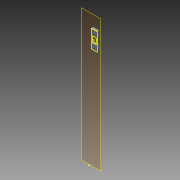
# Autodesk Inventor part: boardHolderv2
Saved by Autodesk Inventor 2014 (Build 180170000, 170)
## iProperties
Created: 2014-01-11
Part Number: boardHolderv2
Material: Generic
Document SubType Name: Modeling
Designer: intern
Density: 1 g/cm^3
Appearance: Default
Author: intern
Autodesk Inventor part; units mm, degrees
ref_plane "YZ Plane" through (0, 0, 0) normal (1, 0, 0) x (0, 1, 0)
ref_plane "XZ Plane" through (0, 0, 0) normal (0, 1, 0) x (-1, 0, 0)
ref_plane "XY Plane" through (0, 0, 0) normal (0, 0, 1) x (1, 0, 0)
ref_plane "Work Plane1" through (0, 0, 0) normal (0, 0, 1) x (1, 0, 0)
sketch "Sketch1" plane through (0, 0, 0) normal (0, 0, 1) x (1, 0, 0)
  circle A0 centre (26.9875, 590.55) radius 15.621 projected
  line L0 (11.3665, 606.171) -> (42.6085, 606.171)
  line L1 (42.6085, 606.171) -> (42.6085, 574.929)
  line L2 (42.6085, 574.929) -> (11.3665, 574.929)
  line L3 (11.3665, 574.929) -> (11.3665, 606.171)
  line L4 (11.3665, 606.171) -> (42.6085, 574.929) construction
  line L5 (42.6085, 606.171) -> (11.3665, 574.929) construction
  line L6 (10.8585, 637.921) -> (43.1165, 637.921)
  line L7 (43.1165, 637.921) -> (43.1165, 543.179)
  line L8 (43.1165, 543.179) -> (10.8585, 543.179)
  line L9 (10.8585, 543.179) -> (10.8585, 637.921)
  line L10 (10.8585, 637.921) -> (43.1165, 543.179) construction
  line L11 (43.1165, 637.921) -> (10.8585, 543.179) construction
  line L12 (42.6085, 606.171) -> (43.1165, 606.171)
  line L13 (11.3665, 606.171) -> (10.8585, 606.171)
  line L14 (11.3665, 574.929) -> (10.8585, 574.929)
  line L15 (42.6085, 574.929) -> (43.1165, 574.929)
  point P0 (0, 0)
  dimension "d0" = 32.258
  dimension "d1" = 94.742
  constraints: 32 end point, 5 equal length, 5 perpendicular, 4 midpoint, 4 point on line, 3 horizontal, 1 vertical
  measures "d0" distance of L7.end L8.end
  measures "d1" distance of L6.end L7.end
extrude "Extrusion1" add sketch "Sketch1" along normal blind 5.08 contours L0 L13 L9 L6 L7 L12 | L2 L15 L7 L8 L9 L14
sketch "Sketch2" plane through (0, 0, 5.08) normal (0, 0, 1) x (1, 0, 0)
  line L0 (10.8585, 606.171) -> (43.1165, 606.171) projected
  line L1 (43.1165, 606.171) -> (43.1165, 637.921) projected
  line L2 (43.1165, 637.921) -> (10.8585, 637.921) projected
  circle A0 centre (26.9875, 590.55) radius 8.9481 projected
  line L3 (35.8299, 591.9213) -> (35.0382, 597.0264) projected
  line L4 (35.0382, 597.0264) -> (30.2211, 598.8934) projected
  line L5 (36.6216, 586.8161) -> (35.8299, 591.9213) projected
  line L6 (32.5963, 583.5779) -> (36.6216, 586.8161) projected
  line L7 (28.5709, 580.3397) -> (32.5963, 583.5779) projected
  line L8 (23.7539, 582.2066) -> (28.5709, 580.3397) projected
  line L9 (28.1112, 583.3043) -> (33.8243, 587.9003) projected
  line L10 (33.8243, 587.9003) -> (32.7007, 595.146) projected
  line L11 (32.7007, 595.146) -> (25.8638, 597.7957) projected
  line L12 (25.8638, 597.7957) -> (20.1507, 593.1997) projected
  line L13 (20.1507, 593.1997) -> (21.2743, 585.954) projected
  line L14 (21.2743, 585.954) -> (28.1112, 583.3043) projected
  line L15 (28.5709, 580.3397) -> (18.9368, 584.0736) projected
  line L16 (18.9368, 584.0736) -> (17.3534, 594.2839) projected
  line L17 (17.3534, 594.2839) -> (25.4041, 600.7603) projected
  line L18 (25.4041, 600.7603) -> (35.0382, 597.0264) projected
  line L19 (35.0382, 597.0264) -> (36.6216, 586.8161) projected
  line L20 (36.6216, 586.8161) -> (28.5709, 580.3397) projected
  line L21 (43.1165, 574.929) -> (10.8585, 574.929) projected
  line L22 (10.8585, 574.929) -> (10.8585, 543.179) projected
  line L23 (10.8585, 543.179) -> (43.1165, 543.179) projected
  line L24 (43.1165, 543.179) -> (43.1165, 574.929) projected
  line L25 (43.1165, 637.921) -> (37.3198, 637.921)
  line L26 (37.3198, 543.179) -> (43.1165, 543.179)
  line L27 (43.1165, 543.179) -> (43.1165, 637.921)
  line L28 (10.8585, 543.179) -> (16.6552, 543.179)
  line L29 (16.6552, 637.921) -> (10.8585, 637.921)
  line L30 (10.8585, 637.921) -> (10.8585, 543.179)
  line L31 (37.3198, 637.921) -> (16.6552, 637.921)
  line L32 (16.6552, 637.921) -> (16.6552, 606.171)
  line L33 (16.6552, 606.171) -> (37.3198, 606.171)
  line L34 (37.3198, 606.171) -> (37.3198, 637.921)
  line L35 (37.3198, 574.929) -> (16.6552, 574.929)
  line L36 (16.6552, 574.929) -> (16.6552, 543.179)
  line L37 (16.6552, 543.179) -> (37.3198, 543.179)
  line L38 (37.3198, 543.179) -> (37.3198, 574.929)
  circle A1 centre (26.9875, 590.55) radius 10.9728
  line L39 (37.3198, 606.171) -> (37.3198, 594.2439)
  line L40 (37.3198, 586.8561) -> (37.3198, 574.929)
  line L41 (43.1165, 637.921) -> (43.1165, 543.179)
  line L42 (43.1165, 543.179) -> (37.3198, 543.179)
  line L43 (37.3198, 637.921) -> (43.1165, 637.921)
  line L44 (16.6552, 637.921) -> (16.6552, 594.2439)
  line L45 (16.6552, 586.8561) -> (16.6552, 543.179)
  line L46 (10.8585, 543.179) -> (43.1165, 543.179)
  line L47 (43.1165, 543.179) -> (43.1165, 574.929)
  line L48 (43.1165, 574.929) -> (10.8585, 574.929)
  line L49 (10.8585, 574.929) -> (10.8585, 543.179)
  line L50 (10.8585, 637.921) -> (43.1165, 637.921)
  line L51 (43.1165, 637.921) -> (43.1165, 606.171)
  line L52 (43.1165, 606.171) -> (10.8585, 606.171)
  line L53 (10.8585, 606.171) -> (10.8585, 637.921)
  line L54 (16.6552, 574.929) -> (10.8585, 574.929)
  line L55 (10.8585, 574.929) -> (10.8585, 543.179)
  line L56 (10.8585, 543.179) -> (16.6552, 543.179)
  line L57 (16.6552, 543.179) -> (16.6552, 574.929)
  line L58 (43.1165, 574.929) -> (37.3198, 574.929)
  line L59 (37.3198, 574.929) -> (37.3198, 543.179)
  line L60 (37.3198, 543.179) -> (43.1165, 543.179)
  line L61 (43.1165, 543.179) -> (43.1165, 574.929)
  line L62 (16.6552, 586.8561) -> (16.6552, 574.929)
  line L63 (16.6552, 574.929) -> (10.8585, 574.929)
  line L64 (10.8585, 574.929) -> (10.8585, 606.171)
  line L65 (10.8585, 606.171) -> (16.6552, 606.171)
  line L66 (16.6552, 606.171) -> (16.6552, 594.2439)
  line L67 (37.3198, 574.929) -> (37.3198, 586.8561)
  line L68 (37.3198, 594.2439) -> (37.3198, 606.171)
  line L69 (43.1165, 606.171) -> (37.3198, 606.171)
  line L70 (43.1165, 606.171) -> (43.1165, 574.929)
  line L71 (43.1165, 574.929) -> (37.3198, 574.929)
  line L72 (43.1165, 574.929) -> (10.8585, 574.929)
  point P0 (0, 0)
  dimension "d4" = 21.9456
  constraints: 96 end point, 16 parallel, 14 perpendicular, 8 collinear, 8 horizontal, 4 point on circle, 4 point on line, 4 vertical, 1 centre point
  measures "d4" diameter of A1
extrude "Extrusion3" add sketch "Sketch2" along normal blind 6.0706 contours L30 L2 L32 L0 | L0 L44 A1 L45 L21 L30 | L32 L2 L34 L0 | L21 L36 L23 L22 | L34 L2 L1 L0 | L0 L27 L21 L40 A1 L39 | L21 L38 L23 L36 | L21 L24 L23 L38
sketch "Sketch4" plane through (0, 0, 11.1506) normal (0, 0, 1) x (1, 0, 0)
  line L0 (37.3198, 606.171) -> (37.3198, 594.2439) projected
  arc A0 (37.3198, 586.8561) -> (37.3198, 594.2439) centre (26.9875, 590.55) ccw projected
  line L1 (37.3198, 586.8561) -> (37.3198, 574.929) projected
  line L2 (37.3198, 574.929) -> (16.6552, 574.929) projected
  line L3 (16.6552, 574.929) -> (16.6552, 586.8561) projected
  arc A1 (16.6552, 594.2439) -> (16.6552, 586.8561) centre (26.9875, 590.55) ccw projected
  line L4 (16.6552, 594.2439) -> (16.6552, 606.171) projected
  line L5 (16.6552, 606.171) -> (37.3198, 606.171) projected
  line L6 (46.9875, 570.55) -> (6.9875, 570.55)
  line L7 (6.9875, 570.55) -> (6.9875, 610.55)
  line L8 (6.9875, 610.55) -> (46.9875, 610.55)
  line L9 (46.9875, 610.55) -> (46.9875, 570.55)
  line L10 (46.9875, 570.55) -> (6.9875, 610.55) construction
  line L11 (6.9875, 570.55) -> (46.9875, 610.55) construction
  line L12 (16.0147, 580.8925) -> (37.9603, 580.8925)
  line L13 (37.9603, 580.8925) -> (37.9603, 600.2075)
  line L14 (37.9603, 600.2075) -> (16.0147, 600.2075)
  line L15 (16.0147, 600.2075) -> (16.0147, 580.8925)
  line L16 (40.4875, 575.55) -> (13.4875, 575.55)
  line L17 (11.9875, 577.05) -> (11.9875, 604.05)
  line L18 (13.4875, 605.55) -> (40.4875, 605.55)
  line L19 (41.9875, 604.05) -> (41.9875, 577.05)
  line L20 (41.9875, 575.55) -> (11.9875, 605.55) construction
  line L21 (11.9875, 575.55) -> (41.9875, 605.55) construction
  circle A2 centre (11.9875, 605.55) radius 1.5
  circle A3 centre (11.9875, 575.55) radius 1.5
  circle A4 centre (41.9875, 575.55) radius 1.5
  circle A5 centre (41.9875, 605.55) radius 1.5
  line L22 (37.9603, 610.55) -> (16.0147, 610.55)
  line L23 (16.0147, 610.55) -> (16.0147, 600.2075)
  line L24 (16.0147, 600.2075) -> (37.9603, 600.2075)
  line L25 (37.9603, 600.2075) -> (37.9603, 610.55)
  circle A6 centre (11.9875, 575.55) radius 1.5
  circle A7 centre (11.9875, 605.55) radius 1.5
  circle A8 centre (41.9875, 605.55) radius 1.5
  circle A9 centre (41.9875, 575.55) radius 1.5
  point P0 (0, 0)
  dimension "d14" = 3
  dimension "d9" = 40
  dimension "d10" = 40
  dimension "d11" = 30
  dimension "d12" = 30
  dimension "d13" = 3
  dimension "d15" = 3
  dimension "d16" = 3
  constraints: 40 end point, 8 coincident, 8 parallel, 6 centre point, 6 horizontal, 6 point on circle, 4 midpoint, 4 perpendicular, 3 vertical, 1 concentric, 1 horizontal alignment, 1 point on line, 1 vertical alignment, 4 other
  measures "d9" distance of L7.end L8.end
  measures "d10" distance of L6.end L7.end
  measures "d11" distance of L20.end L21.end
  measures "d12" distance of L21.start L20.end
  measures "d13" diameter of A2
  measures "d15" diameter of A4
  measures "d16" diameter of A5
extrude "Extrusion5" add sketch "Sketch4" along normal blind 4.4 contours L25 L8 L9 L6 L7 L23 L18 A2 L17 A3 L16 L3 L2 L1 A4 L19 A5 | L18 A5 L19 A4 L16 L1 L12 L13 L25 | L23 L15 L12 L3 L16 A3 L17 A2 L18
sketch "Sketch5" plane through (0, 0, 15.5506) normal (0, 0, 1) x (1, 0, 0)
  circle A0 centre (11.9875, 605.55) radius 1.5 projected
  circle A1 centre (11.9875, 575.55) radius 1.5 projected
  circle A2 centre (41.9875, 575.55) radius 1.5 projected
  circle A3 centre (41.9875, 605.55) radius 1.5 projected
  circle A4 centre (11.9875, 575.55) radius 1.5
  circle A5 centre (41.9875, 575.55) radius 1.5
  circle A6 centre (41.9875, 605.55) radius 1.5
  circle A7 centre (11.9875, 605.55) radius 1.5
  point P0 (0, 0)
  constraints: 4 centre point, 4 coincident, 4 concentric
extrude "Extrusion6" cut sketch "Sketch5" against normal through all
sketch "Sketch6" plane through (10.8585, 543.179, 0) normal (-1, 0, 0) x (0, 0, 1)
  line L0 (11.1506, 31.3834) -> (0, 31.3834) projected
  line L1 (11.1506, 31.3834) -> (11.1506, 27.371) projected
  line L2 (5.08, 33.3586) -> (11.1506, 33.3586) projected
  line L3 (0, 63.3586) -> (11.1506, 63.3586) projected
  line L4 (11.1506, 61.3834) -> (5.08, 61.3834) projected
  line L5 (15.5506, 63.871) -> (15.5506, 60.871) projected
  line L6 (15.5506, 33.871) -> (15.5506, 30.871) projected
  line L7 (11.1506, 31.3834) -> (11.1506, 33.3586)
  line L8 (11.1506, 33.3586) -> (11.1506, 31.3834)
  line L9 (11.1506, 32.371) -> (11.1506, 35.546)
  line L10 (11.1506, 32.371) -> (11.1506, 29.196)
  line L11 (11.1506, 29.196) -> (6.5786, 29.196)
  line L12 (6.5786, 29.196) -> (6.5786, 35.546)
  line L13 (11.1506, 61.3834) -> (11.1506, 63.3586)
  line L14 (11.1506, 62.371) -> (11.1506, 65.546)
  line L15 (11.1506, 65.546) -> (11.1506, 59.196)
  line L16 (11.1506, 27.371) -> (11.1506, 0) projected
  line L17 (6.5786, 35.546) -> (11.1506, 35.546)
  line L18 (11.1506, 65.546) -> (6.5786, 65.546)
  line L19 (6.5786, 65.546) -> (6.5786, 59.196)
  line L20 (6.5786, 59.196) -> (11.1506, 59.196)
  point P0 (0, -543.179)
  dimension "d23" = 3.175
  dimension "d25" = 3.175
  dimension "d26" = 4.572
  dimension "d27" = 3.175
  dimension "d28" = 6.35
  constraints: 26 end point, 4 collinear, 4 parallel, 3 perpendicular, 2 midpoint, 1 point on line
  measures "d23" distance of L9.start L9.end
  measures "d25" distance of L9.start L10.end
  measures "d26" distance of L10.end L11.end
  measures "d27" distance of L14.start L14.end
  measures "d28" distance of L14.end L15.end
extrude "Extrusion7" cut sketch "Sketch6" against normal blind 7.62
sketch "Sketch7" plane through (43.1165, 576.5376, 5.08) normal (1, 0, 0) x (0, 0, -1)
  line L0 (-6.0706, 0) -> (-6.0706, 28.0248) projected
  line L1 (5.08, -1.9752) -> (-6.0706, -1.9752) projected
  line L2 (-6.0706, -5.9876) -> (-6.0706, 34.0124) projected
  line L3 (-6.0706, 30) -> (5.08, 30) projected
  line L4 (-6.0706, 30) -> (-6.0706, 28.0248)
  line L5 (-6.0706, 29.0124) -> (-6.0706, 25.8374)
  line L6 (-6.0706, 25.8374) -> (-6.0706, 32.1874)
  line L7 (-6.0706, -1.9752) -> (-6.0706, 0)
  line L8 (-6.0706, -0.9876) -> (-6.0706, 2.1874)
  line L9 (-6.0706, 2.1874) -> (-6.0706, -0.9876)
  line L10 (-6.0706, -0.9876) -> (-6.0706, -4.1626)
  line L11 (-6.0706, 30) -> (-6.0706, 34.0124) projected
  line L12 (-6.0706, -4.1626) -> (-1.4986, -4.1626)
  line L13 (-1.4986, -4.1626) -> (-1.4986, 2.1874)
  line L14 (-1.4986, 2.1874) -> (-6.0706, 2.1874)
  line L15 (-6.0706, 32.1874) -> (-1.4986, 32.1874)
  line L16 (-1.4986, 32.1874) -> (-1.4986, 25.8374)
  line L17 (-1.4986, 25.8374) -> (-6.0706, 25.8374)
  point P0 (5.08, -576.5376)
  point P1 (-0.4953, -1.9752)
  dimension "d31" = 3.175
  dimension "d32" = 6.35
  dimension "d33" = 3.175
  dimension "d34" = 3.175
  dimension "d37" = 4.572
  constraints: 26 end point, 4 perpendicular, 3 midpoint, 3 parallel, 1 collinear, 6 other
  measures "d31" distance of L5.start L5.end
  measures "d32" distance of L5.end L6.end
  measures "d33" distance of L8.start L8.end
  measures "d34" distance of L8.start L10.end
  measures "d37" distance of L10.end L12.end
extrude "Extrusion8" cut sketch "Sketch7" against normal blind 7.62
sketch "Sketch8" plane through (0, 0, 11.1506) normal (0, 0, 1) x (1, 0, 0)
  line L0 (28.2838, 557.9644) -> (25.6912, 555.7646)
  circle A0 centre (26.9875, 556.8645) radius 1.7
  line L1 (35.4965, 608.725) -> (37.9603, 608.725) projected
  line L2 (37.9603, 608.725) -> (37.9603, 610.55) projected
  line L3 (37.9603, 610.55) -> (43.1165, 610.55) projected
  line L4 (43.1165, 610.55) -> (43.1165, 637.921) projected
  line L5 (43.1165, 637.921) -> (10.8585, 637.921) projected
  line L6 (10.8585, 637.921) -> (10.8585, 610.55) projected
  line L7 (10.8585, 610.55) -> (16.0147, 610.55) projected
  line L8 (16.0147, 610.55) -> (16.0147, 608.725) projected
  line L9 (16.0147, 608.725) -> (18.4785, 608.725) projected
  line L10 (18.4785, 608.725) -> (18.4785, 606.171) projected
  line L11 (18.4785, 606.171) -> (35.4965, 606.171) projected
  line L12 (35.4965, 606.171) -> (35.4965, 608.725) projected
  circle A1 centre (26.9875, 624.2355) radius 1.7
  line L13 (10.8585, 637.921) -> (25.6912, 625.3354)
  line L14 (28.2838, 623.1356) -> (43.1165, 610.55)
  line L15 (43.1165, 637.921) -> (28.2838, 625.3354)
  line L16 (25.6912, 623.1356) -> (10.8585, 610.55)
  point P0 (0, 0)
  dimension "d38" = 3.4
  dimension "d39" = 3.4
  constraints: 10 end point, 6 point on circle, 2 centre point, 2 parallel, 1 midpoint
  measures "d38" diameter of A0
  measures "d39" diameter of A1
extrude "Extrusion10" cut sketch "Sketch8" against normal through all contours A0 L0 | L0 A0 | A1
body "Solid1"
